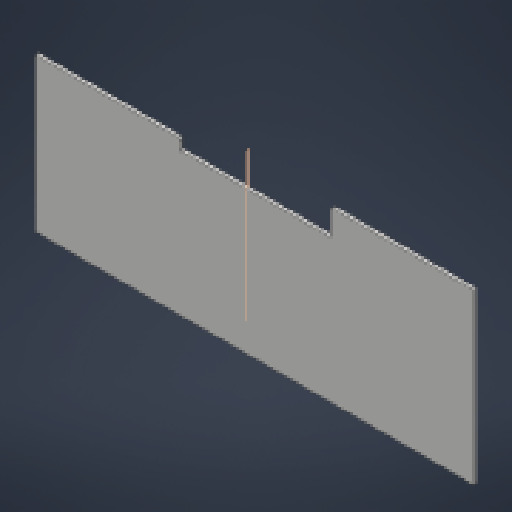
# Autodesk Inventor part: 弹舱1
Saved by Autodesk Inventor 2025 (Build 290162000, 162)
## iProperties
Created: 2025-12-21
Part Number: 弹舱1
Material: 常规
Document SubType Name: Modeling
Designer: XH
Density: 1 g/cm^3
Appearance: 默认
Author: XH
Autodesk Inventor part; units mm, degrees
ref_plane "YZ Plane" through (0, 0, 0) normal (1, 0, 0) x (0, 1, 0)
ref_plane "XZ Plane" through (0, 0, 0) normal (0, 1, 0) x (-1, 0, 0)
ref_plane "XY Plane" through (0, 0, 0) normal (0, 0, 1) x (1, 0, 0)
sketch "草图1" plane through (0, 0, 0) normal (0, 0, 1) x (1, 0, 0)
  line L0 (100, -65) -> (-100, -65)
  line L1 (-100, -65) -> (-100, 65)
  line L2 (-100, 65) -> (100, 65)
  line L3 (100, 65) -> (100, -65)
  line L4 (100, -65) -> (-100, 65) construction
  line L5 (-100, -65) -> (100, 65) construction
  point P0 (0, 0)
  dimension "d0" = 200
  dimension "d1" = 130
  constraints: 12 end point, 2 midpoint, 2 parallel, 1 horizontal, 1 perpendicular
  measures "d0" distance of L1.end L2.end
  measures "d1" distance of L2.end L0.start
extrude "拉伸1" add sketch "草图1" along normal blind 3
sketch "草图2" plane through (-100, 65, 0) normal (0, 1, 0) x (1, 0, 0)
  line L0 (17.9183, -213.0122) -> (17.9183, 66.9878) projected
  line L1 (179.0997, -213.0122) -> (179.0997, 66.9878) projected
  line L2 (37.0997, 66.9878) -> (37.0997, -213.0122) projected
  line L3 (200, 0) -> (0, 0) projected
  line L4 (0, 0) -> (0, -3) projected
  line L5 (200, -3) -> (0, -3) projected
  line L6 (200, 0) -> (200, -3) projected
  line L7 (181.0997, -213.0122) -> (181.0997, 66.9878)
  line L8 (35.0997, 66.9878) -> (35.0997, -213.0122)
  point P0 (100, 0)
  point P1 (181.0997, -3)
  point P2 (181.0997, 0)
  point P3 (35.0997, 0)
  point P4 (35.0997, -3)
  dimension "d4" = 2
  dimension "d5" = 2
  constraints: 4 end point, 2 parallel
  measures "d4" distance between parallel lines of L1 L7
  measures "d5" distance between parallel lines of L2 L8
extrude "拉伸2" cut sketch "草图2" against normal blind 25 contours L8 L3 L2 L5 | L2 L3 L1 L5 | L1 L3 L7 L5
fillet "圆角1" radius 2 2 edges at (81.0997, 65, 1.5) (-64.9003, 65, 1.5)
sketch "草图3" plane through (100, -65, 0) normal (1, 0, 0) x (0, 0, -1)
  line L0 (0, 0) -> (0, 130) projected
  line L1 (0, 130) -> (-3, 130) projected
  line L2 (-3, 0) -> (-3, 130) projected
  line L3 (0, 0) -> (-3, 0) projected
  point P0 (0, 65)
ref_plane "工作平面1" through (0, -65, 0) normal (1, 0, 0) x (0, 0, -1)
extrude "拉伸3" add sketch "草图3" along normal blind 120
mirror "镜像1" about plane through (0, -65, 0) normal (1, 0, 0) of "拉伸3"
sketch "草图4" plane through (0, 0, 0) normal (0, 0, -1) x (-1, 0, 0)
  point P0 (0, 0)
sketch "草图5" plane through (0, 0, 0) normal (0, 0, -1) x (-1, 0, 0)
  line L0 (-220, -65) -> (220, -65) projected
  line L1 (-220, -65) -> (220, -65)
  line L2 (220, -65) -> (220, -99)
  line L3 (220, -99) -> (-220, -99)
  line L4 (-220, -99) -> (-220, -65)
  line L5 (206.0817, -99) -> (-221.9183, -99) projected
  point P0 (0, 0)
  constraints: 8 end point, 2 parallel, 1 collinear, 1 horizontal, 1 perpendicular
extrude "拉伸4" add sketch "草图5" against normal up to surface (3 mm away)
move faces "移动1" translate (15, 0, 0) faces at (-220, -44.3333, 1)
move faces "移动2" translate (0, -15, 0) faces at (-158.9668, 65, 1) (174.3666, 65, 1)
